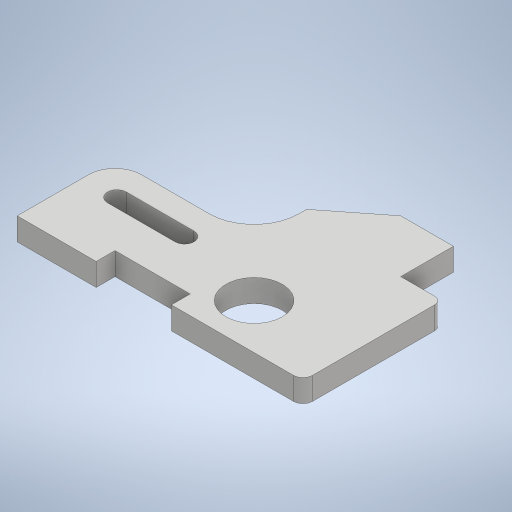
# Autodesk Inventor part: Activity_3_kumar
Saved by Autodesk Inventor 2024 (Build 280153000, 153)
## iProperties
Created: 2024-09-25
Part Number: Activity_3_kumar
Material: Generic
Document SubType Name: Modeling
Designer: itsimg
Density: 1 g/cm^3
Appearance: Default
Author: itsimg
Autodesk Inventor part; units mm, degrees
ref_plane "YZ Plane" through (0, 0, 0) normal (1, 0, 0) x (0, 1, 0)
ref_plane "XZ Plane" through (0, 0, 0) normal (0, 1, 0) x (-1, 0, 0)
ref_plane "XY Plane" through (0, 0, 0) normal (0, 0, 1) x (1, 0, 0)
sketch "Sketch1" plane through (0, 0, 0) normal (0, 0, 1) x (1, 0, 0)
  line L0 (23.0088, 62.2159) -> (23.0088, 24.2159)
  line L1 (175.0088, 29.2159) -> (175.0088, 94.2159)
  line L2 (97.0088, 104.2159) -> (97.0088, 100.2159)
  line L3 (73.0088, 76.2159) -> (37.0088, 76.2159)
  line L4 (97.0088, 104.2159) -> (125.0088, 126.2159)
  line L5 (23.0088, 24.2159) -> (65.0088, 24.2159)
  line L6 (65.0088, 24.2159) -> (65.0088, 34.2159)
  line L7 (65.0088, 34.2159) -> (105.0088, 34.2159)
  line L8 (105.0088, 34.2159) -> (105.0088, 24.2159)
  line L9 (105.0088, 24.2159) -> (170.0088, 24.2159)
  line L10 (125.0088, 126.2159) -> (153.0088, 126.2159)
  line L11 (153.0088, 98.2159) -> (171.0088, 98.2159)
  arc A0 (37.0088, 76.2159) -> (23.0088, 62.2159) centre (37.0088, 62.2159) ccw
  arc A1 (73.0088, 76.2159) -> (97.0088, 100.2159) centre (73.0088, 100.2159) ccw
  arc A2 (175.0088, 94.2159) -> (171.0088, 98.2159) centre (171.0088, 94.2159) ccw
  arc A3 (170.0088, 24.2159) -> (175.0088, 29.2159) centre (170.0088, 29.2159) ccw
  circle A4 centre (125.0088, 48.2159) radius 15
  line L12 (153.0088, 126.2159) -> (153.0088, 98.2159)
  line L13 (41.0088, 64.2159) -> (77.0088, 64.2159)
  line L14 (77.0088, 54.2159) -> (41.0088, 54.2159)
  arc A5 (41.0088, 64.2159) -> (41.0088, 54.2159) centre (41.0088, 59.2159) ccw
  arc A6 (77.0088, 54.2159) -> (77.0088, 64.2159) centre (77.0088, 59.2159) ccw
  point P0 (0, 0)
  point P1 (23.0088, 76.2159)
  point P2 (175.0088, 24.2159)
  point P3 (175.0088, 98.2159)
  dimension "d0" = 52
  dimension "d5" = 74
  dimension "d7" = 102
  dimension "d8" = 80
  dimension "d9" = 102
  dimension "d11" = 42
  dimension "d12" = 82
  dimension "d13" = 152
  dimension "d14" = 74
  dimension "d15" = 14
  dimension "d16" = 24
  dimension "d17" = 4
  dimension "d18" = 5
  dimension "d30" = 30
  dimension "d31" = 24
  dimension "d32" = 102
  dimension "d33" = 10
  dimension "d34" = 23.0088
  dimension "d35" = 24.2159
  dimension "d38" = 130
  dimension "d42" = 5
  dimension "d43" = 18
  dimension "d44" = 54
  dimension "d45" = 35
  dimension "d46" = 5
  constraints: 30 end point, 12 point on circle, 11 tangent, 7 centre point, 7 point on line, 6 perpendicular, 4 horizontal, 2 parallel, 2 vertical
  measures "d0" distance of point (23.009, 76.216) L0.end
  measures "d5" distance of point (175.009, 24.216) point (175.009, 98.216)
  measures "d7" distance from line of L9 L10.end
  measures "d8" distance from line of L5 L2.start
  measures "d9" distance from line of L0 L4.end
  measures "d11" distance of L5.end L0.end
  measures "d12" distance of L8.end L0.end
  measures "d13" distance of point (175.009, 24.216) L0.end
  measures "d14" horizontal distance of point (23.009, 76.216) L2.start
  measures "d15" radius of A0
  measures "d16" radius of A1
  measures "d17" radius of A2
  measures "d18" radius of A3
  measures "d30" diameter of A4
  measures "d31" distance from line of L9 A4.centre
  measures "d32" distance from line of L0 A4.centre
  measures "d33" distance of L5.end L6.end
  measures "d34" distance from line of point (0, 0) L0
  measures "d35" distance from line of point (0, 0) L5
  measures "d38" distance between parallel lines of L0 L12
  measures "d42" radius of A5
  measures "d43" distance from line of L0 A5.centre
  measures "d44" distance from line of L0 A6.centre
  measures "d45" distance from line of L5 A5.centre
  measures "d46" radius of A6
extrude "Extrusion1" add sketch "Sketch1" along normal blind 12
body "Solid1"
